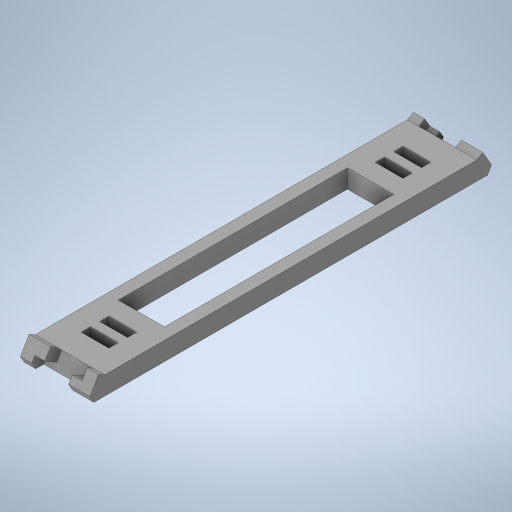
# Autodesk Inventor part: base
Saved by Autodesk Inventor 2024.3 (Build 283343000, 343)
## iProperties
Created: 2024-10-09
Part Number: base
Material: Generic
Document SubType Name: Modeling
Designer: pjcaa
Density: 1 g/cm^3
Appearance: Default(2)
Author: pjcaa
Autodesk Inventor part; units mm, degrees
ref_plane "YZ Plane" through (0, 0, 0) normal (1, 0, 0) x (0, 1, 0)
ref_plane "XZ Plane" through (0, 0, 0) normal (0, 1, 0) x (-1, 0, 0)
ref_plane "XY Plane" through (0, 0, 0) normal (0, 0, 1) x (1, 0, 0)
sketch "Sketch1" plane through (0, 0, 0) normal (0, 0, 1) x (1, 0, 0)
  line L0 (-85, -15) -> (85, -15)
  line L1 (85, -15) -> (85, 15)
  line L2 (85, 15) -> (-85, 15)
  line L3 (-85, 15) -> (-85, -15)
  line L4 (-85, -15) -> (85, 15) construction
  line L5 (85, -15) -> (-85, 15) construction
  point P0 (0, 0)
  dimension "d0" = 170
  dimension "d1" = 30
  constraints: 12 end point, 2 midpoint, 2 parallel, 1 horizontal, 1 perpendicular
  measures "d0" distance of L2.end L1.end
  measures "d1" distance of L1.end L0.end
extrude "Extrusion1" add sketch "Sketch1" along normal blind 8
sketch "Sketch2" plane through (-85, 15, 0) normal (0, 1, 0) x (1, 0, 0)
  line L0 (170, 0) -> (0, 0) construction
  line L1 (0, 0) -> (0, -8) construction
  line L2 (170, -8) -> (0, -8) construction
  line L3 (170, 0) -> (170, -8) construction
  line L4 (0, -8) -> (0, 0)
  line L5 (85, 0) -> (85, -8) construction
  line L6 (0, 0) -> (4.6188, -8)
  line L7 (0, -8) -> (4.6188, -8)
  line L8 (170, -8) -> (170, 0)
  line L9 (170, 0) -> (165.3812, -8)
  line L10 (170, -8) -> (165.3812, -8)
  point P0 (1.7321, 0)
  dimension "d7" = 30
  constraints: 14 end point, 2 collinear, 2 point on line, 1 midpoint, 1 symmetric about line
  measures "d7" angle of L1 L6
extrude "Extrusion3" cut sketch "Sketch2" against normal through all
sketch "Sketch3" plane through (-85, -15, 0) normal (-0.866, 0, 0.5) x (0.5, 0, 0.866)
  line L0 (9.2376, 0) -> (0, 0) construction
  line L1 (9.2376, 30) -> (9.2376, 0) construction
  line L2 (0, 30) -> (9.2376, 30) construction
  line L3 (0, 30) -> (0, 0) construction
  line L4 (9.2376, 30) -> (0, 30)
  line L5 (9.2376, 30) -> (9.2376, 20.7624)
  line L6 (0, 0) -> (9.2376, 0)
  line L7 (0, 0) -> (0, 9.2376)
  line L8 (9.2376, 30) -> (9.2376, 0) projected
  line L9 (9.2376, 20.7624) -> (4.3376, 20.7624)
  line L10 (4.3376, 20.7624) -> (4.3376, 25.1)
  line L11 (4.3376, 25.1) -> (0, 25.1)
  line L12 (0, 30) -> (0, 25.1)
  line L13 (0, 9.2376) -> (4.9, 9.2376)
  line L14 (4.9, 9.2376) -> (4.9, 4.9)
  line L15 (4.9, 4.9) -> (9.2376, 4.9)
  line L16 (9.2376, 0) -> (9.2376, 4.9)
  point P0 (42.5, 15)
  point P1 (4.6188, 30)
  point P2 (9.2376, 15)
  point P3 (4.6188, 30)
  point P4 (9.2376, 15)
  dimension "d15" = 4.9
  dimension "d16" = 4.9
  dimension "d17" = 4.9
  dimension "d18" = 4.9
  constraints: 24 end point, 7 perpendicular, 4 midpoint, 4 point on line, 3 collinear, 2 horizontal
  measures "d15" distance of L5.end L9.end
  measures "d16" distance between parallel lines of L2 L11
  measures "d17" distance between parallel lines of L0 L15
  measures "d18" distance of L7.end L13.end
extrude "Extrusion4" add sketch "Sketch3" along normal blind 3
sketch "Sketch4" plane through (-85, -5.7624, 0) normal (-0.866, 0, 0.5) x (0.5, 0, 0.866)
  line L0 (4.9, -4.3376) -> (9.2376, -4.3376) projected
  line L1 (9.2376, 11.5248) -> (9.2376, -4.3376) projected
  line L2 (9.2376, 11.5248) -> (4.3376, 11.5248) projected
  line L3 (4.3376, 11.5248) -> (4.3376, 15.8624) projected
  line L4 (4.3376, 15.8624) -> (0, 15.8624) projected
  line L5 (0, 15.8624) -> (0, 0) projected
  line L6 (0, 0) -> (4.9, 0) projected
  line L7 (4.9, 0) -> (4.9, -4.3376) projected
  point P0 (42.5, 5.7624)
extrude "Extrusion5" cut sketch "Sketch4" against normal blind 3
sketch "Sketch6" plane through (85, -15, 0) normal (0.866, 0, 0.5) x (0.5, 0, -0.866)
  line L0 (0, 0) -> (-9.2376, 0) construction
  line L1 (0, 0) -> (0, 30) construction
  line L2 (-9.2376, 30) -> (0, 30) construction
  line L3 (-9.2376, 0) -> (-9.2376, 30) construction
  line L4 (0, 0) -> (-9.2376, 0)
  line L5 (-9.2376, 0) -> (-9.2376, 9.2376)
  line L6 (-9.2376, 9.2376) -> (-4.3376, 9.2376)
  line L7 (-4.3376, 9.2376) -> (-4.3376, 4.9)
  line L8 (-4.3376, 4.9) -> (0, 4.9)
  line L9 (0, 0) -> (0, 4.9)
  line L10 (0, 0) -> (0, 30) projected
  line L11 (0, 30) -> (-9.2376, 30)
  line L12 (-9.2376, 25.1) -> (-9.2376, 30)
  line L13 (-9.2376, 25.1) -> (-4.9, 25.1)
  line L14 (-4.9, 25.1) -> (-4.9, 20.7624)
  line L15 (-4.9, 20.7624) -> (0, 20.7624)
  line L16 (0, 20.7624) -> (0, 30)
  point P0 (-42.5, 15)
  point P1 (-7.0688, 25.1)
  dimension "d24" = 4.9
  dimension "d25" = 4.9
  dimension "d26" = 4.9
  dimension "d27" = 4.9
  constraints: 24 end point, 7 perpendicular, 4 collinear, 4 point on line, 2 horizontal, 1 midpoint
  measures "d24" distance between parallel lines of L1 L14
  measures "d25" distance from line of L11 point (-7.069, 25.1)
  measures "d26" distance of L5.end L6.end
  measures "d27" distance between parallel lines of L0 L8
extrude "Extrusion7" add sketch "Sketch6" along normal blind 3
sketch "Sketch7" plane through (85, -10.1, 0) normal (0.866, 0, 0.5) x (0.5, 0, -0.866)
  line L0 (-4.9, 20.2) -> (-9.2376, 20.2) projected
  line L1 (-9.2376, 4.3376) -> (-9.2376, 20.2) projected
  line L2 (-9.2376, 4.3376) -> (-4.3376, 4.3376) projected
  line L3 (-4.3376, 4.3376) -> (-4.3376, 0) projected
  line L4 (-4.3376, 0) -> (0, 0) projected
  line L5 (0, 0) -> (0, 15.8624) projected
  line L6 (0, 15.8624) -> (-4.9, 15.8624) projected
  line L7 (-4.9, 15.8624) -> (-4.9, 20.2) projected
  point P0 (-42.5, 10.1)
extrude "Extrusion8" cut sketch "Sketch7" against normal blind 3
sketch "Sketch5" plane through (-85, -15, 0) normal (0, -1, 0) x (1, 0, 0)
  line L0 (4.6188, 8) -> (165.3812, 8) construction
  line L1 (4.6188, 8) -> (2.0207, 9.5) construction
  line L2 (-2.5981, 1.5) -> (2.0207, 9.5) construction
  line L3 (0, 0) -> (-2.5981, 1.5) construction
  line L4 (0, 0) -> (170, 0) construction
  line L5 (0, 0) -> (-2.5981, 1.5)
  line L6 (-1.7321, 3) -> (-2.5981, 1.5)
  line L7 (0, 0) -> (-1.7321, 3)
  line L8 (170, 0) -> (172.5981, 1.5) projected
  line L9 (167.9793, 9.5) -> (172.5981, 1.5) projected
  line L10 (165.3812, 8) -> (167.9793, 9.5) projected
  line L11 (170, 0) -> (171.7321, 3)
  line L12 (171.7321, 3) -> (172.5981, 1.5)
  line L13 (172.5981, 1.5) -> (170, 0)
  point P0 (85, 0)
  dimension "d21" = 30
  dimension "d32" = 30
  constraints: 12 end point, 2 point on line, 1 perpendicular
  measures "d21" angle of L7 L3
  measures "d32" angle of L8 L11
extrude "Extrusion6" cut sketch "Sketch5" against normal through all
sketch "Sketch9" plane through (0, 0, 8) normal (0, 0, 1) x (1, 0, 0)
  line L0 (80.3812, -15) -> (80.3812, -5.7624) construction
  line L1 (80.3812, -5.7624) -> (80.3812, 10.1) construction
  line L2 (80.3812, 10.1) -> (80.3812, 15) construction
  line L3 (80.3812, 15) -> (-80.3812, 15) construction
  line L4 (-80.3812, 15) -> (-80.3812, 5.7624) construction
  line L5 (-80.3812, 5.7624) -> (-80.3812, -10.1) construction
  line L6 (-80.3812, -10.1) -> (-80.3812, -15) construction
  line L7 (-80.3812, -15) -> (80.3812, -15) construction
  line L8 (49.5, -10) -> (-49.5, -10)
  line L9 (-49.5, -10) -> (-49.5, 10)
  line L10 (-49.5, 10) -> (49.5, 10)
  line L11 (49.5, 10) -> (49.5, -10)
  line L12 (49.5, -10) -> (-49.5, 10) construction
  line L13 (-49.5, -10) -> (49.5, 10) construction
  line L14 (73.5, -10) -> (53.5, -10) construction
  line L15 (53.5, -10) -> (53.5, 10) construction
  line L16 (53.5, 10) -> (73.5, 10) construction
  line L17 (73.5, 10) -> (73.5, -10) construction
  line L18 (63.5, -10) -> (63.5, 10) construction
  line L19 (53.5, 0) -> (73.5, 0) construction
  line L20 (69.5, -6) -> (57.5, -6) construction
  line L21 (57.5, -6) -> (57.5, 6) construction
  line L22 (57.5, 6) -> (69.5, 6) construction
  line L23 (69.5, 6) -> (69.5, -6) construction
  line L24 (69.5, -6) -> (57.5, 6) construction
  line L25 (57.5, -6) -> (69.5, 6) construction
  line L26 (69.5, -6) -> (65.5, -6)
  line L27 (65.5, -6) -> (65.5, 6)
  line L28 (65.5, 6) -> (69.5, 6)
  line L29 (69.5, 6) -> (69.5, -6)
  line L30 (57.5, -6) -> (61.5, -6)
  line L31 (61.5, -6) -> (61.5, 6)
  line L32 (61.5, 6) -> (57.5, 6)
  line L33 (57.5, 6) -> (57.5, -6)
  line L34 (0, -10) -> (0, 10) construction
  line L35 (-69.5, -6) -> (-57.5, -6) construction
  line L36 (-57.5, -6) -> (-57.5, 6) construction
  line L37 (-57.5, 6) -> (-69.5, 6) construction
  line L38 (-69.5, 6) -> (-69.5, -6) construction
  line L39 (-69.5, -6) -> (-57.5, 6) construction
  line L40 (-57.5, -6) -> (-69.5, 6) construction
  line L41 (-69.5, -6) -> (-65.5, -6)
  line L42 (-65.5, -6) -> (-65.5, 6)
  line L43 (-65.5, 6) -> (-69.5, 6)
  line L44 (-69.5, 6) -> (-69.5, -6)
  line L45 (-57.5, -6) -> (-61.5, -6)
  line L46 (-61.5, -6) -> (-61.5, 6)
  line L47 (-61.5, 6) -> (-57.5, 6)
  line L48 (-57.5, 6) -> (-57.5, -6)
  point P0 (0, 0)
  point P1 (49.5, 0)
  point P2 (63.5, 0)
  point P3 (-63.5, 0)
  dimension "d53" = 99
  dimension "d54" = 20
  dimension "d55" = 20
  dimension "d56" = 20
  dimension "d57" = 4
  dimension "d58" = 12
  dimension "d60" = 4
  dimension "d61" = 12
  dimension "d62" = 4
  dimension "d63" = 12
  constraints: 82 end point, 12 midpoint, 11 symmetric about line, 10 parallel, 6 perpendicular, 5 horizontal, 1 horizontal alignment
  measures "d53" distance of L9.end L10.end
  measures "d54" distance of L8.end L9.end
  measures "d55" distance of L15.end L16.end
  measures "d56" distance of L14.end L15.end
  measures "d57" distance between parallel lines of L11 L15
  measures "d58" distance of L21.end L22.end
  measures "d60" distance of L27.end L28.end
  measures "d61" distance of L26.end L27.end
  measures "d62" distance of L32.end L31.end
  measures "d63" distance of L31.end L30.end
extrude "Extrusion10" cut sketch "Sketch9" against normal through all
body "Solid1"
